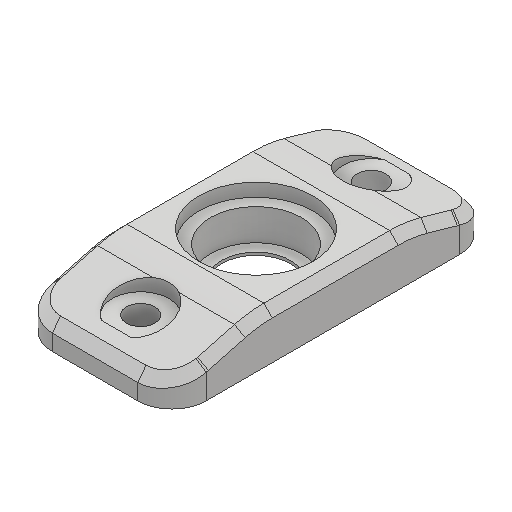
# Autodesk Inventor part: 3DP_ABS_Z_Axis_Ball_Screw_Thrust_Bearing_Block
Saved by Autodesk Inventor 2026.1 (Build 301233000, 233)
## iProperties
Created: 2016-10-08
Part Number: 3DP_ABS_Z_Axis_Ball_Screw_Thrust_Bearing_Block
Material: Ogólny
Document SubType Name: Modeling
Designer: Andrzej
Density: 1 g/cm^3
Appearance: Domyślna
Author: Andrzej
Autodesk Inventor part; units mm, degrees
ref_plane "YZ Plane" through (0, 0, 0) normal (1, 0, 0) x (0, 1, 0)
ref_plane "XZ Plane" through (0, 0, 0) normal (0, 1, 0) x (-1, 0, 0)
ref_plane "XY Plane" through (0, 0, 0) normal (0, 0, 1) x (1, 0, 0)
sketch "Szkic1" plane through (0, 0, 0) normal (0, 0, 1) x (1, 0, 0)
  line L0 (-12.7879, 23.1455) -> (14.2121, 23.1455)
  line L1 (14.2121, 23.1455) -> (14.2121, -33.3545)
  line L2 (14.2121, -33.3545) -> (-12.7879, -33.3545)
  line L3 (-12.7879, -33.3545) -> (-12.7879, 23.1455)
  circle A0 centre (0.7121, -5.1045) radius 8
  point P0 (0.7121, 15.1455)
  point P1 (0.7121, -25.3545)
  dimension "d4" = 27
  dimension "d5" = 56.5
  dimension "d6" = 28.25
  dimension "d7" = 13.5
  dimension "d8" = 13.5
  dimension "d9" = 13.5
  dimension "d10" = 8
  dimension "d11" = 8
  dimension "d12" = 16
  constraints: 8 end point, 2 parallel, 1 centre point, 1 coincident, 1 horizontal, 1 perpendicular
  measures "d4" distance of L1.end L2.end
  measures "d5" distance of L0.end L1.end
  measures "d6" distance from line of L2 point (0.712, -5.104)
  measures "d7" distance from line of L3 point (0.712, -5.104)
  measures "d8" distance from line of L3 point (0.712, -25.354)
  measures "d9" distance from line of L3 point (0.712, 15.146)
  measures "d10" distance from line of L0 point (0.712, 15.146)
  measures "d11" distance from line of point (0.712, -25.354) L2
  measures "d12" diameter of A0
extrude "Wyciągnięcie proste1" add sketch "Szkic1" along normal blind 5.5
sketch "Szkic2" plane through (0, 0, 0) normal (0, 0, -1) x (-1, 0, 0)
  circle A0 centre (-0.7121, -5.1045) radius 8 projected
  line L0 (12.7879, 23.1455) -> (-14.2121, 23.1455) projected
  line L1 (-14.2121, 23.1455) -> (-14.2121, -33.3545) projected
  line L2 (-14.2121, -33.3545) -> (12.7879, -33.3545) projected
  line L3 (12.7879, -33.3545) -> (12.7879, 23.1455) projected
  circle A1 centre (-0.7121, -5.1045) radius 6
  point P0 (0, 0)
  dimension "d16" = 12
  constraints: 1 centre point, 1 coincident
  measures "d16" diameter of A1
extrude "Wyciągnięcie proste2" add sketch "Szkic2" along normal blind 0.5 contours A0 | L3 L2 L1 L0
sketch "Szkic3" plane through (0, 0, 5.5) normal (0, 0, 1) x (1, 0, 0)
  circle A0 centre (0.7121, -5.1045) radius 8 projected
  line L0 (14.2121, 23.1455) -> (-12.7879, 23.1455) projected
  line L1 (-12.7879, 23.1455) -> (-12.7879, -33.3545) projected
  line L2 (-12.7879, -33.3545) -> (14.2121, -33.3545) projected
  line L3 (14.2121, -33.3545) -> (14.2121, 23.1455) projected
  circle A1 centre (0.7121, -5.1045) radius 10
  point P0 (0, 0)
  dimension "d19" = 20
  constraints: 1 centre point, 1 coincident
  measures "d19" diameter of A1
extrude "Wyciągnięcie proste3" add sketch "Szkic3" along normal blind 2.3 contours L3 L2 L1 L0
chamfer "Faza1" distance 15 distance2 4 1 edges at (0.7121, -33.3545, 7.8) measured on face at (1.1139, 17.0379, 7.8)
chamfer "Faza2" distance 14 distance2 4 1 edges at (0.7121, 23.1455, 7.8) measured on face at (0.3103, 17.0379, 7.8)
fillet "Zaokrąglenie1" radius 6 4 edges at (-12.7879, -33.3545, 1.65) (-12.7879, 23.1455, 1.65) (14.2121, 23.1455, 1.65) (14.2121, -33.3545, 1.65)
fillet "Zaokrąglenie2" radius 20 2 edges at (0.7121, -18.3545, 7.8) (0.7121, 9.1455, 7.8)
hole "Otwór1" at (0.7121, 15.1455, 0) at (0.7121, -25.3545, 0) direction (0, 0, 1) diameter 5 depth 8
hole "Otwór2" at (0.7121, -25.3545, 0) at (0.7121, 15.1455, 0) direction (0, 0, -1) diameter 5 depth 8
sketch "Szkic4" plane through (0, 0, 7.8) normal (0, 0, 1) x (1, 0, 0)
  circle A0 centre (0.7121, -25.3545) radius 2.5 projected
  circle A1 centre (0.7121, 15.1455) radius 2.5 projected
  circle A2 centre (0.7121, -25.3545) radius 5
  circle A3 centre (0.7121, 15.1455) radius 5
  point P0 (0, 0)
  dimension "d44" = 10
  dimension "d45" = 10
  constraints: 2 centre point, 2 coincident
  measures "d44" diameter of A2
  measures "d45" diameter of A3
extrude "Wyciągnięcie proste4" cut sketch "Szkic4" against normal blind 3
chamfer "Faza3" distance 1.5 angle 45 16 edges at (14.2121, 14.4922, 6.2724) (12.4547, 21.3882, 4.3021) (0.7121, 23.1455, 3.8) (-11.0306, 21.3882, 4.3021) (-12.7879, 14.4922, 6.2724) (-12.7879, 9.1185, 7.6067) (-12.7879, -4.6946, 7.8) (-12.7879, -18.3322, 7.6305) (-12.7879, -24.1206, 6.2623) (-11.0306, -31.5971, 4.2686) (0.7121, -33.3545, 3.8) (12.4547, -31.5971, 4.2686) (14.2121, -24.1206, 6.2623) (14.2121, -18.3322, 7.6305) (14.2121, -4.6946, 7.8) (14.2121, 9.1185, 7.6067)
equation "\"d6\" = 0.5 * d5"
equation "\"d7\" = 0.5 * d4"
equation "\"d8\" = d7"
equation "\"d9\" = d7"
equation "\"d10\" = d11"
